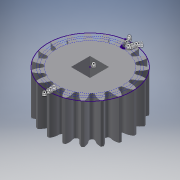
# Autodesk Inventor part: gear 1 shaft
Saved by Autodesk Inventor 2017 (Build 210142000, 142)
## iProperties
Created: 2018-04-17
Part Number: gear 1 shaft
Material: Generic
Document SubType Name: Modeling
Designer: RKL
Density: 1 g/cm^3
Appearance: Default
Author: RKL
Autodesk Inventor part; units mm, degrees
ref_plane "YZ Plane" through (0, 0, 0) normal (1, 0, 0) x (0, 1, 0)
ref_plane "XZ Plane" through (0, 0, 0) normal (0, 1, 0) x (-1, 0, 0)
ref_plane "XY Plane" through (0, 0, 0) normal (0, 0, 1) x (1, 0, 0)
sketch "Sketch1" plane through (0, 0, 0) normal (0, 0, 1) x (1, 0, 0)
  spline S0 degree 3 poles (-2.891, 20.8) (-2.7137, 20.5767) (-2.359, 20.13) (-1.9026, 19.4044) (-1.5895, 18.7631) (-1.39, 18.2274) (-1.3359, 17.9472) (-1.3089, 17.8071) knots 0 0 0 0 0.085522 0.171036 0.256527 0.299287 0.342003 0.342003 0.342003 0.342003
  spline S1 degree 3 poles (-1.3089, 17.8071) (-1.2897, 17.6125) (-1.261, 17.3204) (-1.1397, 16.9483) (-1.0079, 16.6856) (-0.8203, 16.4576) (-0.5788, 16.2868) (-0.2935, 16.1974) (0, 16.2127) (0.2935, 16.1974) (0.5788, 16.2868) (0.8203, 16.4576) (1.0079, 16.6856) (1.1397, 16.9483) (1.261, 17.3204) (1.2897, 17.6125) (1.3089, 17.8071) knots 0 0 0 0 0.058444 0.087678 0.116921 0.146138 0.175348 0.204525 0.233777 0.263029 0.292205 0.321415 0.350633 0.379875 0.40911 0.467554 0.467554 0.467554 0.467554
  spline S2 degree 3 poles (1.3089, 17.8071) (1.3359, 17.9472) (1.39, 18.2274) (1.5895, 18.7631) (1.9026, 19.4044) (2.359, 20.13) (2.7137, 20.5767) (2.891, 20.8) knots 0 0 0 0 0.042716 0.085476 0.170967 0.256481 0.342003 0.342003 0.342003 0.342003
  circle A0 centre (0, 0) radius 16.2076 construction
  circle A1 centre (0, 0) radius 17.8542 construction
  circle A2 centre (0, 0) radius 19 construction
  circle A3 centre (0, 0) radius 21
  point P0 (-2.3716, 20.1207)
  point P1 (-1.916, 19.397)
  point P2 (-1.5439, 18.6273)
  point P3 (-1.4014, 18.2242)
  point P4 (-1.2238, 17.2289)
  point P5 (-1.1329, 16.9511)
  point P6 (-0.9985, 16.6913)
  point P7 (-0.8112, 16.4671)
  point P8 (-0.5714, 16.3003)
  point P9 (-0.2924, 16.2149)
  point P10 (0, 16.2076)
  point P11 (0.2924, 16.2149)
  point P12 (0.5714, 16.3003)
  point P13 (0.8112, 16.4671)
  point P14 (0.9985, 16.6913)
  point P15 (1.1329, 16.9511)
  point P16 (1.2238, 17.2289)
  point P17 (1.4014, 18.2242)
  point P18 (1.5439, 18.6273)
  point P19 (1.916, 19.397)
  point P20 (2.3716, 20.1207)
  constraints: 4 centre point, 2 point on circle, 57 other
extrude "Extrusion1" add sketch "Sketch1" against normal blind 20
extrude "Extrusion2" cut sketch "Sketch1" against normal through all contours A3 S2 S1 S0 picked at (0.3069, 19.4328)
pattern_circular "Circular Pattern1" count 19 over 360 about axis through (0, 0, 0) along (0, 0, -1) of "Extrusion2"
sketch "Sketch2" plane through (0, 0, 0) normal (0, 0, 1) x (1, 0, 0)
  line L0 (4.7625, -4.7625) -> (-4.7625, -4.7625)
  line L1 (-4.7625, -4.7625) -> (-4.7625, 4.7625)
  line L2 (-4.7625, 4.7625) -> (4.7625, 4.7625)
  line L3 (4.7625, 4.7625) -> (4.7625, -4.7625)
  line L4 (4.7625, -4.7625) -> (-4.7625, 4.7625) construction
  line L5 (-4.7625, -4.7625) -> (4.7625, 4.7625) construction
  point P0 (0, 0)
  dimension "d7" = 9.525
  constraints: 12 end point, 2 midpoint, 2 parallel, 2 perpendicular, 1 horizontal
  measures "d7" distance of L0.end L1.end
extrude "Extrusion3" cut sketch "Sketch2" against normal through all
equation "\"d0\" = FaceWidth"
equation "\"Module\" = 2"
equation "\"PressureAngle\" = 20deg"
equation "\"UnitProfileClearance\" = 0.25"
equation "\"UnitRoundRadius\" = 0.3335"
equation "\"HeadDiameter\" = 42"
equation "\"RootDiameter\" = 32.41524"
equation "\"BaseDiameter\" = 35.70832"
equation "\"PitchDiameter\" = 38"
equation "\"FaceWidth\" = 20"
equation "\"HelixAngle\" = 0"
equation "\"UnitCorrection\" = 0"
equation "\"UnitAddendumModification\" = 0"
equation "\"CircularPitch\" = 6.283185"
equation "\"UnitBacklashShift\" = -0.14619"
equation "\"TotalToolShift\" = -0.29238"
equation "\"IsInternal\" = 0"
body "Solid1"
